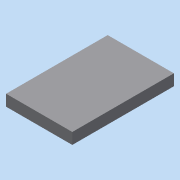
# Autodesk Inventor part: breadboard lol
Saved by Autodesk Inventor 2015 (Build 190159000, 159)
## iProperties
Created: 2015-06-24
Part Number: breadboard lol
Material: Generic
Document SubType Name: Modeling
Designer: Rahul
Density: 1 g/cm^3
Appearance: Default
Author: Rahul
Autodesk Inventor part; units mm, degrees
ref_plane "YZ Plane" through (0, 0, 0) normal (1, 0, 0) x (0, 1, 0)
ref_plane "XZ Plane" through (0, 0, 0) normal (0, 1, 0) x (-1, 0, 0)
ref_plane "XY Plane" through (0, 0, 0) normal (0, 0, 1) x (1, 0, 0)
sketch "Sketch1" plane through (0, 0, 0) normal (0, 1, 0) x (-1, 0, 0)
  line L0 (24.9059, -36.2412) -> (-30.0241, -36.2412)
  line L1 (-30.0241, -36.2412) -> (-30.0241, 48.0688)
  line L2 (-30.0241, 48.0688) -> (24.9059, 48.0688)
  line L3 (24.9059, 48.0688) -> (24.9059, -36.2412)
  point P0 (0, 0)
  dimension "d0" = 84.31
  dimension "d1" = 54.93
  constraints: 8 end point, 2 parallel, 1 horizontal, 1 perpendicular
  measures "d0" distance of L0.end L1.end
  measures "d1" distance of L0.start L0.end
extrude "Extrusion1" add sketch "Sketch1" against normal blind 9.3
body "Solid1"
